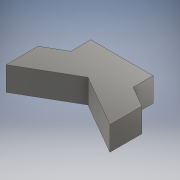
# Autodesk Inventor part: Łapka
Saved by Autodesk Inventor 2017 (Build 210142000, 142)
## iProperties
Created: 2018-05-29
Part Number: Łapka
Material: Stainless Steel, Austenitic
Document SubType Name: Modeling
Designer: Pies
Density: 8 g/cm^3
Appearance: Semi-Polished
Author: Pies
Autodesk Inventor part; units mm, degrees
ref_plane "YZ Plane" through (0, 0, 0) normal (1, 0, 0) x (0, 1, 0)
ref_plane "XZ Plane" through (0, 0, 0) normal (0, 1, 0) x (-1, 0, 0)
ref_plane "XY Plane" through (0, 0, 0) normal (0, 0, 1) x (1, 0, 0)
sketch "Sketch1" plane through (0, 0, 0) normal (0, 0, 1) x (1, 0, 0)
  line L0 (0, -8.5) -> (12.9904, -16)
  line L1 (12.9904, -16) -> (12.9904, -8)
  line L2 (0, -8.5) -> (-12.9904, -16)
  line L3 (-12.9904, -16) -> (-12.9904, -8)
  line L4 (-7.7942, 0) -> (7.7942, 0)
  line L5 (-12.9904, -8) -> (-7.7942, -5)
  line L6 (-7.7942, -5) -> (-7.7942, 0)
  line L7 (12.9904, -8) -> (7.7942, -5)
  line L8 (7.7942, -5) -> (7.7942, 0)
  point P0 (0, 0)
  constraints: 18 end point, 2 perpendicular, 2 vertical, 1 horizontal
extrude "Extrusion1" add sketch "Sketch1" along normal blind 6
sketch "Sketch2" plane through (-7.7942, 0, 0) normal (0, 1, 0) x (1, 0, 0)
  line L0 (15.5885, 0) -> (15.5885, -6) construction
  line L1 (15.5885, -3) -> (0, -3) construction
  line L2 (0, 0) -> (0, -6) construction
  point P0 (7.7942, 0)
  point P1 (11.5885, -3)
  point P2 (4, -3)
  constraints: 2 end point, 2 midpoint, 2 point on line
hole "Hole2" at (3.7942, 0, 3) at (-3.7942, 0, 3) direction (0, -1, 0) diameter 3.2 depth 5 clearance for "Hex Head Cap Screw ISO 24017" size "M3" standard "ISO"
body "Solid1"
